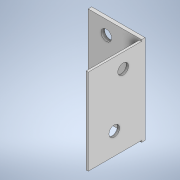
# Autodesk Inventor part: L angle
Saved by Autodesk Inventor 2021 (Build 250183000, 183)
## iProperties
Created: 2023-06-07
Part Number: L angle
Material: Generic
Document SubType Name: Modeling
Designer: badig
Density: 1 g/cm^3
Appearance: Default
Author: badig
Autodesk Inventor part; units mm, degrees
ref_plane "YZ Plane" through (0, 0, 0) normal (1, 0, 0) x (0, 1, 0)
ref_plane "XZ Plane" through (0, 0, 0) normal (0, 1, 0) x (-1, 0, 0)
ref_plane "XY Plane" through (0, 0, 0) normal (0, 0, 1) x (1, 0, 0)
sketch "Sketch1" plane through (0, 0, 0) normal (0, 0, 1) x (1, 0, 0)
  line L0 (-7.9197, 10.2868) -> (-22.9197, 10.2868)
  line L1 (-22.9197, 10.2868) -> (-22.9197, -14.7132)
  line L2 (-22.9197, -14.7132) -> (-7.9197, -14.7132)
  line L3 (-7.9197, -14.7132) -> (-7.9197, 10.2868)
  point P0 (0, 0)
  dimension "d0" = 15
  dimension "d1" = 25
  constraints: 8 end point, 2 parallel, 1 horizontal, 1 perpendicular
  measures "d0" distance of L2.end L1.end
  measures "d1" distance of L1.end L0.end
extrude "Extrusion1" add sketch "Sketch1" along normal blind 1
sketch "Sketch2" plane through (0, 0, 1) normal (0, 0, 1) x (1, 0, 0)
  circle A0 centre (-17.8268, 6.422) radius 2.5
  circle A1 centre (-17.8268, -7.5909) radius 2.5
  point P0 (0, 0)
  dimension "d4" = 5
  dimension "d5" = 5
  constraints: 2 centre point
  measures "d4" diameter of A0
  measures "d5" diameter of A1
hole "Hole1" at (-17.8268, 6.422, 1) at (-17.8268, -7.5909, 1) direction (0, 0, -1) diameter 3 end through all
sketch "Sketch3" plane through (0, 0, 1) normal (0, 0, 1) x (1, 0, 0)
  line L0 (-22.9197, -14.7132) -> (-7.9197, -14.7132) projected
  line L1 (-7.9197, 10.2868) -> (-22.9197, 10.2868) projected
  line L2 (-7.9197, -14.7132) -> (-7.9197, 10.2868) projected
  line L3 (-8.5412, 9.8751) -> (-7.9197, 9.8751)
  line L4 (-7.9197, 9.8751) -> (-7.9197, -14.2385)
  line L5 (-7.9197, -14.2385) -> (-8.5412, -14.2385)
  line L6 (-8.5412, -14.2385) -> (-8.5412, 9.8751)
  point P0 (0, 0)
  dimension "d13" = 25
  dimension "d14" = 15
  constraints: 8 end point, 2 parallel, 1 horizontal, 1 perpendicular, 1 point on line
  measures "d13" distance between parallel lines of L0 L1
  measures "d14" distance of L1.start L1.end
extrude "Extrusion2" add sketch "Sketch3" along normal blind 15
sketch "Sketch4" plane through (-8.5412, -14.2385, 1) normal (-1, 0, 0) x (0, 0, 1)
  circle A0 centre (5.1833, 19.9887) radius 2.5
  circle A1 centre (7.6833, 6.1285) radius 2.5
  point P0 (-1, 14.2385)
  dimension "d17" = 5
  dimension "d18" = 5
  constraints: 2 centre point
  measures "d17" diameter of A0
  measures "d18" diameter of A1
hole "Hole2" at (-8.5412, 5.7501, 6.1833) at (-8.5412, -8.1101, 8.6833) direction (1, 0, 0) diameter 3 end through all
body "Solid1"
